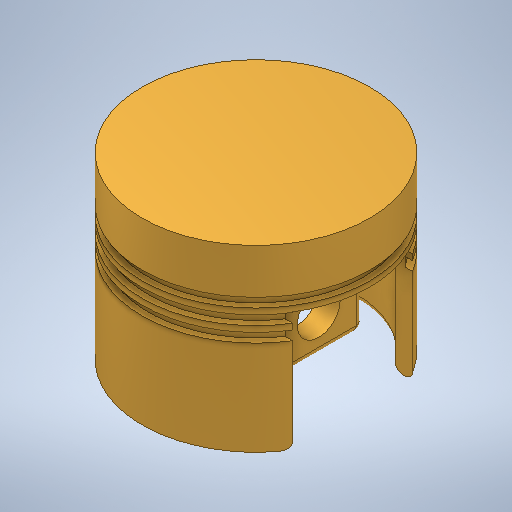
# Autodesk Inventor part: Piston2
Saved by Autodesk Inventor 2025.1 (Build 291241000, 241)
## iProperties
Created: 2024-07-30
Part Number: Piston2
Material: Generic
Document SubType Name: Modeling
Designer: vedan
Density: 1 g/cm^3
Appearance: Brass - Satin
Author: vedan
Autodesk Inventor part; units mm, degrees
ref_plane "YZ Plane" through (0, 0, 0) normal (1, 0, 0) x (0, 1, 0)
ref_plane "XZ Plane" through (0, 0, 0) normal (0, 1, 0) x (-1, 0, 0)
sketch "Sketch1" plane through (0, 0, 0) normal (0, 0, 1) x (1, 0, 0)
  line L0 (29.4, -6.5532) -> (122.4832, -6.5532) construction
  line L1 (46.5416, 12.9723) -> (46.5416, 55.2013) construction
  line L2 (29.4, 29.9576) -> (61.15, 29.9576)
  line L3 (61.3825, -20.0424) -> (61.15, -20.0424)
  line L4 (57.15, -20.0424) -> (61.3825, -20.0424)
  line L5 (29.4, 42.3483) -> (29.4, -56.369) construction
  line L6 (29.4, 29.9576) -> (29.4, 24.4639)
  line L7 (29.4, 21.5715) -> (29.4, 18.6327)
  line L8 (29.4, 15.2385) -> (29.4, 13.3085)
  line L9 (29.4, 29.9576) -> (29.4, 15.2385)
  line L10 (61.15, 29.9576) -> (59.375, 29.9576)
  line L11 (59.375, 17.4133) -> (61.15, 17.4133)
  line L12 (59.375, 17.4133) -> (59.375, 14.8137)
  line L13 (59.375, 14.8137) -> (61.15, 14.8137)
  line L14 (61.15, 13.1714) -> (59.375, 13.1714)
  line L15 (59.375, 13.1714) -> (59.375, 10.5719)
  line L16 (59.375, 10.5719) -> (61.15, 10.5719)
  line L17 (61.15, 8.9299) -> (59.375, 8.9299)
  line L18 (59.375, 8.9299) -> (59.375, 6.3303)
  line L19 (59.375, 6.3303) -> (61.15, 6.3303)
  line L20 (61.15, 29.9576) -> (61.15, 17.4133)
  line L21 (61.15, 14.8137) -> (61.15, 13.1714)
  line L22 (61.15, 10.5719) -> (61.15, 8.9299)
  line L23 (61.15, 6.3303) -> (61.15, -20.0424)
  line L24 (57.15, 13.3085) -> (29.4, 13.3085)
  line L25 (57.15, -20.0424) -> (57.15, 13.3085)
  point P0 (0, 0)
  point P1 (57.15, -6.5532)
  dimension "d4" = 31.75
  dimension "d15" = 50
  dimension "d17" = 4
  dimension "d65" = 1.6423
  dimension "d66" = 1.642
  constraints: 52 end point, 9 perpendicular, 8 vertical, 6 point on line, 3 collinear, 3 horizontal
  measures "d4" distance of L2.end L2.start
  measures "d15" distance of L2.end L3.end
  measures "d17" distance of L3.end L4.start
  measures "d65" distance of L14.start L13.end
  measures "d66" distance of L17.start L16.end
revolve "Revolution2" add sketch "Sketch1" angle 360 about axis through (29.4, 42.3483, 0) along (0, -1, 0)
ref_plane "Work Plane9" through (31.75, 0, 0) normal (1, 0, 0) x (0, 1, 0)
sketch "Sketch18" plane through (31.75, 0, 0) normal (1, 0, 0) x (0, 1, 0)
  line L0 (-20.0424, 31.75) -> (-20.0424, -31.75) construction
  line L1 (-20.0424, 31.75) -> (-20.0424, 16.75) construction
  line L2 (-20.0424, -31.75) -> (-20.0424, -16.75) construction
  line L3 (-20.0424, 16.75) -> (13.3085, 16.75) construction
  line L4 (13.3085, 27.75) -> (13.3085, -27.75) construction
  line L5 (-20.0424, -16.75) -> (13.3085, -16.75) construction
  line L6 (-20.0424, 16.75) -> (13.3085, 16.75)
  line L7 (13.3085, 16.75) -> (13.3085, -16.75)
  line L8 (13.3085, -16.75) -> (-20.0424, -16.75)
  line L9 (-20.0424, -16.75) -> (-20.0424, 16.75)
  point P0 (0, 0)
  dimension "d68" = 15
  dimension "d69" = 15
  constraints: 16 end point, 4 point on line, 3 horizontal, 2 parallel, 1 perpendicular
  measures "d68" distance of L0.start L1.end
  measures "d69" distance of L0.end L2.end
extrude "Extrusion6" cut sketch "Sketch18" along normal through all both and the other way through all
sketch "Sketch19" plane through (0, 0, 0) normal (0, 1, 0) x (-1, 0, 0)
  arc A0 (-7.2754, 16.75) -> (-51.5246, 16.75) centre (-29.4, 0) ccw construction
  point P0 (0, 0)
ref_plane "Work Plane8" through (29.4, 21.633, 0) normal (0, -1, 0) x (1, 0, 0)
sketch "Sketch20" plane through (29.4, 21.633, 0) normal (0, -1, 0) x (1, 0, 0)
  arc A0 (26.9722, 16.75) -> (-26.9722, 16.75) centre (0, 0) ccw construction
  line L0 (-31.75, 0) -> (31.75, 0) construction
  line L1 (0, 0) -> (17.5, 0) construction
  line L2 (11.5, 12.5) -> (17.5, 12.5)
  line L3 (17.5, 12.5) -> (17.5, -12.5)
  line L4 (17.5, -12.5) -> (11.5, -12.5)
  line L5 (11.5, 12.5) -> (11.5, -12.5)
  arc A1 (24.8583, 16.75) -> (-24.8583, 16.75) centre (0, 0) ccw construction
  line L6 (-11.5, 12.5) -> (-17.5, 12.5)
  line L7 (-17.5, 12.5) -> (-17.5, -12.5)
  line L8 (-17.5, -12.5) -> (-11.5, -12.5)
  line L9 (-11.5, 12.5) -> (-11.5, -12.5)
  point P0 (-29.4, 0)
  point P1 (17.1094, 0)
  point P2 (-11.5, 0)
  point P3 (17.5, 0)
  dimension "d73" = 25
  dimension "d95" = 35
  dimension "d96" = 23
  constraints: 20 end point, 2 horizontal, 2 point on circle, 2 point on line, 1 midpoint, 1 parallel, 1 perpendicular, 1 vertical
  measures "d73" distance of L2.end L3.end
  measures "d95" distance of L7.start L2.end
  measures "d96" distance of L6.start L2.start
extrude "Extrusion7" add sketch "Sketch20" along normal blind 32
fillet "Fillet13" radius 2 2 edges at (29.4, -20.0424, -31.75) (29.4, -20.0424, -27.75)
fillet "Fillet17" radius 2 24 edges at (40.9, 1.4708, 12.5) (43.9, -10.367, 12.5) (46.9, 1.4708, 12.5) (40.9, 1.4708, -12.5) (40.9, -10.367, 0) (46.9, -10.367, 0) (46.9, 1.4708, -12.5) (43.9, -10.367, -12.5) (17.9, 1.4708, 12.5) (17.9, -10.367, 0) (17.9, 1.4708, -12.5) (11.9, 1.4708, 12.5) (14.9, -10.367, 12.5) (14.9, -10.367, -12.5) (11.9, 1.4708, -12.5) (11.9, -10.367, 0) (17.9, 13.3085, 0) (14.9, 13.3085, 12.5) (11.9, 13.3085, 0) (14.9, 13.3085, -12.5) (40.9, 13.3085, 0) (43.9, 13.3085, -12.5) (43.9, 13.3085, 12.5) (46.9, 13.3085, 0)
fillet "Fillet19" radius 2 2 edges at (53.9484, -20.0424, 16.75) (4.8516, -20.0424, 16.75)
sketch "Sketch23" plane through (46.9, -8.367, 10.5) normal (1, 0, 0) x (0, 0, -1)
  circle A0 centre (10.5, 8.367) radius 6
  dimension "d97" = 12
  constraints: 1 centre point, 1 coincident
  measures "d97" diameter of A0
extrude "Extrusion9" cut sketch "Sketch23" against normal through all
body "Solid1"
